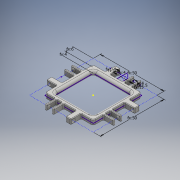
# Autodesk Inventor part: square
Saved by Autodesk Inventor 2016 (Build 200138000, 138)
## iProperties
Created: 2016-11-12
Part Number: square
Material: Generic
Document SubType Name: Modeling
Designer: Chris
Density: 1 g/cm^3
Appearance: Default
Author: Chris
Autodesk Inventor part; units mm, degrees
sketch "Sketch1" plane through (0, 0, 0) normal (0, 0, 1) x (1, 0, 0)
  line L0 (-25, -25) -> (25, -25) construction
  line L1 (25, -25) -> (25, 25) construction
  line L2 (25, 25) -> (-25, 25) construction
  line L3 (-25, 25) -> (-25, -25) construction
  line L4 (-19, 19) -> (19, 19)
  line L5 (19, 19) -> (19, -19)
  line L6 (19, -19) -> (-19, -19)
  line L7 (-19, -19) -> (-19, 19)
  line L8 (15, 15) -> (-15, 15)
  line L9 (-15, 15) -> (-15, -15)
  line L10 (-15, -15) -> (15, -15)
  line L11 (15, -15) -> (15, 15)
  line L12 (-7.5, 25) -> (7.5, 25) construction
  line L13 (-9.5, 25) -> (-5.5, 25) construction
  line L14 (5.5, 25) -> (9.5, 25) construction
  line L15 (5.5, 25) -> (4, 25) construction
  line L16 (9.5, 25) -> (11, 25) construction
  point P0 (0, 0)
  point P1 (-25, 0)
  point P2 (0, 25)
  point P3 (-7.5, 25)
  point P4 (7.5, 25)
  dimension "d2" = 50
  dimension "d3" = 50
  dimension "d4" = 6
  dimension "d5" = 4
  dimension "d6" = 15
  dimension "d9" = 4
  dimension "d10" = 4
  dimension "d11" = 1.5
  constraints: 34 end point, 8 coincident, 6 horizontal, 6 parallel, 5 midpoint, 3 perpendicular, 1 collinear, 1 horizontal alignment, 1 vertical alignment, 6 other
  measures "d2" distance of L2.end L1.end
  measures "d3" distance of L1.end L0.end
  measures "d4" distance between parallel lines of L4 L2
  measures "d5" distance between parallel lines of L8 L4
  measures "d6" distance of L12.start L12.end
  measures "d9" distance of L13.start L13.end
  measures "d10" distance of L14.start L14.end
  measures "d11" distance of L14.end L16.end
extrude "Extrusion1" add sketch "Sketch1" along normal mid plane 4
ref_plane "Work Plane1" through (-9.5, 25, 0) normal (1, 0, 0) x (0, 1, 0)
ref_plane "Work Plane2" through (-5.5, 25, 0) normal (1, 0, 0) x (0, 1, 0)
ref_plane "Work Plane3" through (4, 25, 0) normal (1, 0, 0) x (0, 1, 0)
ref_plane "Work Plane4" through (5.5, 25, 0) normal (1, 0, 0) x (0, 1, 0)
ref_plane "Work Plane5" through (9.5, 25, 0) normal (1, 0, 0) x (0, 1, 0)
ref_plane "Work Plane6" through (11, 25, 0) normal (1, 0, 0) x (0, 1, 0)
sketch "Sketch2" plane through (0, 0, 0) normal (1, 0, 0) x (0, 1, 0)
  line L0 (19, -2) -> (19, 2) projected
  line L1 (19, 2) -> (19, -2) projected
  line L2 (19, 2) -> (27, 2)
  line L3 (27, 2) -> (27, -2)
  line L4 (27, -2) -> (19, -2)
  line L5 (19, -2) -> (19, 2)
  circle A0 centre (25, 0) radius 2 construction
  point P0 (0, 0)
  constraints: 8 end point, 2 parallel, 2 tangent, 1 centre point, 1 coincident, 1 horizontal, 1 perpendicular
extrude "Extrusion2" add sketch "Sketch2" against normal up to surface (4 mm away) from surface at -5.5
extrude "Extrusion3" add sketch "Sketch2" along normal up to surface (1.5 mm away) from surface at 4
extrude "Extrusion4" add sketch "Sketch2" along normal up to surface (1.5 mm away) from surface at 9.5
sketch "Sketch3" plane through (0, 0, 0) normal (0, 0, 1) x (1, 0, 0)
  line L0 (25, 25) -> (-25, 25) construction
  line L1 (-9.5, 25) -> (-9, 25)
  line L2 (-9.5, 26.5) -> (-9.5, 25)
  line L3 (-5.5, 25) -> (-6, 25)
  line L4 (-5.5, 25) -> (-5.5, 26.5)
  line L5 (5.5, 25) -> (6, 25)
  line L6 (5.5, 25) -> (5.5, 26.5)
  line L7 (9.5, 25) -> (9.5, 26.5)
  line L8 (9.5, 25) -> (9, 25)
  arc A0 (-5.5, 26.5) -> (-6, 25) centre (-3.5, 25) ccw
  arc A1 (-9, 25) -> (-9.5, 26.5) centre (-11.5, 25) ccw
  arc A2 (6, 25) -> (5.5, 26.5) centre (3.5, 25) ccw
  arc A3 (9.5, 26.5) -> (9, 25) centre (11.5, 25) ccw
  point P0 (0, 0)
  dimension "d18" = 3
  dimension "d31" = 0.5
  constraints: 16 end point, 8 point on circle, 4 centre point, 4 equal length, 4 vertical, 3 equal radius, 2 horizontal, 1 point on line, 7 other
  measures "d18" diameter of L2.start L1
  measures "d31" distance of L1.start L1.end
revolve "Revolution1" cut sketch "Sketch3" angle 360 about axis through (25, 25, 0) along (-1, 0, 0) contours L2 A1 L1 | L3 A0 L4
revolve "Revolution2" add sketch "Sketch3" angle 360 about axis through (25, 25, 0) along (-1, 0, 0) contours L6 A2 L5 | L8 A3 L7
pattern_circular "Circular Pattern1" count 4 over 360 about axis through (0, 0, -10) along (0, 0, 1) of "Extrusion2", "Extrusion3", "Extrusion4", "Revolution2", "Revolution1"
fillet "Fillet2" radius 2 8 edges at (-19, 19, 0) (-15, 15, 0) (15, 15, 0) (19, 19, 0) (15, -15, 0) (19, -19, 0) (-15, -15, 0) (-19, -19, 0)
fillet "Fillet3" radius 0.75 48 edges at (-9.5, 19, 0) (-5.5, 19, 0) (4, 19, 0) (5.5, 19, 0) (9.5, 19, 0) (11, 19, 0) (19, 9.5, 0) (19, 5.5, 0) (19, -4, 0) (19, -5.5, 0) (19, -9.5, 0) (19, -11, 0) (9.5, -19, 0) (5.5, -19, 0) (-4, -19, 0) (-5.5, -19, 0) (-9.5, -19, 0) (-11, -19, 0) (-19, -9.5, 0) (-19, -5.5, 0) (-19, 4, 0) (-19, 5.5, 0) (-19, 9.5, 0) (-19, 11, 0) (-27, 11, 0) (-27, 9.5, 0) (-27, 5.5, 0) (-27, 4, 0) (-27, -5.5, 0) (-27, -9.5, 0) (-11, -27, 0) (-9.5, -27, 0) (-5.5, -27, 0) (-4, -27, 0) (5.5, -27, 0) (9.5, -27, 0) (27, -11, 0) (27, -9.5, 0) (27, -5.5, 0) (27, -4, 0) (27, 9.5, 0) (27, 5.5, 0) (11, 27, 0) (9.5, 27, 0) (5.5, 27, 0) (4, 27, 0) (-5.5, 27, 0) (-9.5, 27, 0)
chamfer "Chamfer1" distance 0.4 angle 45 176 edges at (-19, 14.375, -2) (-18.4142, 18.4142, -2) (-13.625, 19, -2) (-9.7197, 19.2197, -2) (-9.5, 23, -2) (-9.2803, 26.7803, -2) (-7.5, 27, -2) (-5.7197, 26.7803, -2) (-5.5, 23, -2) (-5.2803, 19.2197, -2) (-0.75, 19, -2) (3.7803, 19.2197, -2) (4, 23, -2) (4.75, 27, -2) (5.5, 23, -2) (5.7197, 19.2197, -2) (7.5, 19, -2) (9.2803, 19.2197, -2) (9.5, 23, -2) (10.25, 27, -2) (11, 23, -2) (11.2197, 19.2197, -2) (14.375, 19, -2) (18.4142, 18.4142, -2) (19, 13.625, -2) (19.2197, 9.7197, -2) (23, 9.5, -2) (26.7803, 9.2803, -2) (27, 7.5, -2) (26.7803, 5.7197, -2) (23, 5.5, -2) (19.2197, 5.2803, -2) (19, 0.75, -2) (19.2197, -3.7803, -2) (23, -4, -2) (27, -4.75, -2) (23, -5.5, -2) (19.2197, -5.7197, -2) (19, -7.5, -2) (19.2197, -9.2803, -2) (23, -9.5, -2) (27, -10.25, -2) (23, -11, -2) (19.2197, -11.2197, -2) (19, -14.375, -2) (18.4142, -18.4142, -2) (13.625, -19, -2) (9.7197, -19.2197, -2) (9.5, -23, -2) (9.2803, -26.7803, -2) (7.5, -27, -2) (5.7197, -26.7803, -2) (5.5, -23, -2) (5.2803, -19.2197, -2) (0.75, -19, -2) (-3.7803, -19.2197, -2) (-4, -23, -2) (-4.75, -27, -2) (-5.5, -23, -2) (-5.7197, -19.2197, -2) (-7.5, -19, -2) (-9.2803, -19.2197, -2) (-9.5, -23, -2) (-10.25, -27, -2) (-11, -23, -2) (-11.2197, -19.2197, -2) (-14.375, -19, -2) (-18.4142, -18.4142, -2) (-19, -13.625, -2) (-19.2197, -9.7197, -2) (-23, -9.5, -2) (-26.7803, -9.2803, -2) (-27, -7.5, -2) (-26.7803, -5.7197, -2) (-23, -5.5, -2) (-19.2197, -5.2803, -2) (-19, -0.75, -2) (-19.2197, 3.7803, -2) (-23, 4, -2) (-27, 4.75, -2) (-23, 5.5, -2) (-19.2197, 5.7197, -2) (-19, 7.5, -2) (-19.2197, 9.2803, -2) (-23, 9.5, -2) (-27, 10.25, -2) (-23, 11, -2) (-19.2197, 11.2197, -2) (-19, 7.5, 2) (-19.2197, 5.7197, 2) (-23, 5.5, 2) (-27, 4.75, 2) (-23, 4, 2) (-19.2197, 3.7803, 2) (-19, -0.75, 2) (-19.2197, -5.2803, 2) (-23, -5.5, 2) (-26.7803, -5.7197, 2) (-27, -7.5, 2) (-26.7803, -9.2803, 2) (-23, -9.5, 2) (-19.2197, -9.7197, 2) (-19, -13.625, 2) (-18.4142, -18.4142, 2) (-14.375, -19, 2) (-11.2197, -19.2197, 2) (-11, -23, 2) (-10.25, -27, 2) (-9.5, -23, 2) (-9.2803, -19.2197, 2) (-7.5, -19, 2) (-5.7197, -19.2197, 2) (-5.5, -23, 2) (-4.75, -27, 2) (-4, -23, 2) (-3.7803, -19.2197, 2) (0.75, -19, 2) (5.2803, -19.2197, 2) (5.5, -23, 2) (5.7197, -26.7803, 2) (7.5, -27, 2) (9.2803, -26.7803, 2) (9.5, -23, 2) (9.7197, -19.2197, 2) (13.625, -19, 2) (18.4142, -18.4142, 2) (19, -14.375, 2) (19.2197, -11.2197, 2) (23, -11, 2) (27, -10.25, 2) (23, -9.5, 2) (19.2197, -9.2803, 2) (19, -7.5, 2) (19.2197, -5.7197, 2) (23, -5.5, 2) (27, -4.75, 2) (23, -4, 2) (19.2197, -3.7803, 2) (19, 0.75, 2) (19.2197, 5.2803, 2) (23, 5.5, 2) (26.7803, 5.7197, 2) (27, 7.5, 2) (26.7803, 9.2803, 2) (23, 9.5, 2) (19.2197, 9.7197, 2) (19, 13.625, 2) (18.4142, 18.4142, 2) (14.375, 19, 2) (11.2197, 19.2197, 2) (11, 23, 2) (10.25, 27, 2) (9.5, 23, 2) (9.2803, 19.2197, 2) (7.5, 19, 2) (5.7197, 19.2197, 2) (5.5, 23, 2) (4.75, 27, 2) (4, 23, 2) (3.7803, 19.2197, 2) (-0.75, 19, 2) (-5.2803, 19.2197, 2) (-5.5, 23, 2) (-5.7197, 26.7803, 2) (-7.5, 27, 2) (-9.2803, 26.7803, 2) (-9.5, 23, 2) (-9.7197, 19.2197, 2) (-13.625, 19, 2) (-18.4142, 18.4142, 2) (-19, 14.375, 2) (-19.2197, 11.2197, 2) (-23, 11, 2) (-27, 10.25, 2) (-23, 9.5, 2) (-19.2197, 9.2803, 2)
fillet "Fillet4" radius 2 16 edges at (14.4142, -14.4142, -2) (15, 0, -2) (14.4142, 14.4142, -2) (0, 15, -2) (-14.4142, 14.4142, -2) (-15, 0, -2) (-14.4142, -14.4142, -2) (0, -15, -2) (-14.4142, -14.4142, 2) (-15, 0, 2) (-14.4142, 14.4142, 2) (0, 15, 2) (14.4142, 14.4142, 2) (15, 0, 2) (14.4142, -14.4142, 2) (0, -15, 2)
equation "\"d2\" = sidelength"
equation "\"d3\" = sidelength"
equation "\"d4\" = springlength"
equation "\"d5\" = diam"
equation "\"d6\" = matespace"
equation "\"d9\" = fingerwidth - 0.5 * tolerance"
equation "\"d10\" = fingerwidth + 0.5 * tolerance"
equation "\"d11\" = springwidth"
equation "\"d7\" = diam"
equation "\"d12\" = diam"
equation "\"d14\" = diam"
equation "\"d16\" = diam"
equation "\"d18\" = dentdiam"
equation "\"sidelength\" = 50"
equation "\"diam\" = 4"
equation "\"dent\" = 0.5"
equation "\"dentdiam\" = 3"
equation "\"tolerance\" = 0"
equation "\"fingerwidth\" = 4"
equation "\"springwidth\" = 1.5"
equation "\"matespace\" = 15"
equation "\"springlength\" = 6"
body "Solid1"
